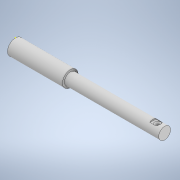
# Autodesk Inventor part: eixo final
Saved by Autodesk Inventor 2022.1 (Build 261234020, 234B)
## iProperties
Created: 2023-08-18
Part Number: eixo final
Material: Generic
Document SubType Name: Modeling
Designer: SENAI
Density: 1 g/cm^3
Appearance: Default
Author: SENAI
Autodesk Inventor part; units mm, degrees
ref_plane "YZ Plane" through (0, 0, 0) normal (1, 0, 0) x (0, 1, 0)
sketch "Sketch1" plane through (0, 0, 0) normal (0, 0, 1) x (1, 0, 0)
  line L0 (0, 0) -> (239, 0)
  line L1 (239, 0) -> (239, 9.5)
  line L2 (0, 0) -> (0, 12.5)
  line L3 (0, 12.5) -> (88, 12.5)
  line L4 (239, 9.5) -> (88, 9.5)
  line L5 (88, 9.5) -> (88, 12.5)
  dimension "d1" = 9.5
  dimension "d3" = 12.5
  dimension "d19" = 88
  dimension "d21" = 151
  constraints: 12 end point, 3 horizontal, 2 perpendicular, 1 vertical
  measures "d1" distance of L0.end L1.end
  measures "d3" distance of L0.start L2.end
  measures "d19" distance of L2.end L3.end
  measures "d21" distance of L1.end L4.end
revolve "Revolution1" add sketch "Sketch1" angle 360 about axis through (0, 0, 0) along (1, 0, 0)
ref_plane "Work Plane3" through (44, 12.5, 0) normal (0, 1, 0) x (-1, 0, 0)
ref_plane "Work Plane4" through (44, 12.5, 0) normal (0, 1, 0) x (-1, 0, 0)
ref_plane "Work Plane5" through (163.5, 9.5, 0) normal (0, 1, 0) x (-1, 0, 0)
sketch "Sketch6" plane through (163.5, 9.5, 0) normal (0, 1, 0) x (-1, 0, 0)
  line L0 (-75.5, 9.5) -> (-75.5, -9.5) projected
  circle A0 centre (-64.5, 0) radius 5
  point P0 (163.5, 0)
  point P1 (-75.5, 0)
  dimension "d27" = 10
  dimension "d28" = 11
  constraints: 1 centre point, 1 midpoint
  measures "d27" diameter of A0
  measures "d28" distance of point (-75.5, 0) A0.centre
extrude "Extrusion5" cut sketch "Sketch6" against normal blind 2
sketch "Sketch7" plane through (228, 7.5, 0) normal (0, 1, 0) x (1, 0, 0)
  circle A0 centre (0, 0) radius 2
  point P0 (-228, 0)
  dimension "d32" = 4
  constraints: 1 centre point
  measures "d32" diameter of A0
extrude "Extrusion6" cut sketch "Sketch7" against normal blind 5
fillet "Fillet2" radius 3.5 1 edges at (226, 7.5, 0)
sketch "Sketch8" plane through (44, 12.5, 0) normal (0, 1, 0) x (-1, 0, 0)
  point P0 (44, 0)
sketch "Sketch9" plane through (163.5, 9.5, 0) normal (0, 1, 0) x (-1, 0, 0)
  circle A0 centre (-64.5, 0) radius 5 projected
  line L0 (-64.5, 5) -> (-56.5, 5)
  line L1 (-64.5, -5) -> (-56.5, -5)
  line L2 (-56.5, -5) -> (-56.5, 5)
  point P0 (163.5, 0)
  dimension "d36" = 8
  dimension "d37" = 8
  constraints: 6 end point, 2 horizontal, 2 point on circle, 2 tangent
  measures "d36" distance of L0.start L0.end
  measures "d37" distance of L1.start L1.end
extrude "Extrusion7" cut sketch "Sketch9" against normal blind 2 contours A0 L0 L2 L1
ref_plane "Work Plane6" through (0, 4.75, 0) normal (0, 1, 0) x (-1, 0, 0)
body "Solid1"
